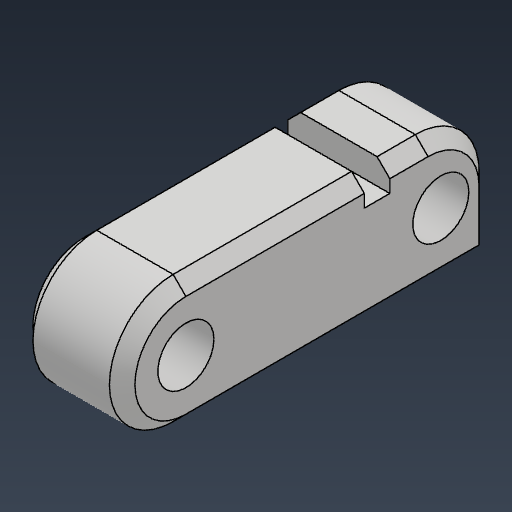
# Autodesk Inventor part: Chipanschlag L2.0
Saved by Autodesk Inventor 2023.1 (Build 271208000, 208)
## iProperties
Part Number: Chipanschlag L2.0
Material: Generisch
Document SubType Name: Modeling
Designer: rYan
Density: 1 g/cm^3
Appearance: Vorgabe
Author: rYan
Autodesk Inventor part; units mm, degrees
ref_plane "YZ Plane" through (0, 0, 0) normal (1, 0, 0) x (0, 1, 0)
ref_plane "XZ Plane" through (0, 0, 0) normal (0, 1, 0) x (-1, 0, 0)
ref_plane "XY Plane" through (0, 0, 0) normal (0, 0, 1) x (1, 0, 0)
sketch "Skizze1" plane through (0, 0, 0) normal (1, 0, 0) x (0, 1, 0)
  line L0 (0, 0) -> (-10, 0) construction
  circle A0 centre (0, 0) radius 1.1
  circle A1 centre (-10, 0) radius 1.1
  arc A2 (-10, 2.5) -> (-10, -2.5) centre (-10, 0) ccw
  line L1 (-10, -2.5) -> (2, -2.5)
  line L2 (-10, 2.5) -> (-0.5, 2.5)
  arc A3 (2, 0) -> (-0.5, 2.5) centre (-0.5, 0) ccw
  line L3 (2, 0) -> (2, -2.5)
  dimension "d0" = 10
  dimension "d1" = 2.2
  dimension "d2" = 2.2
  dimension "d3" = 2.5
  dimension "d8" = 2.5
  dimension "d9" = 2
  constraints: 8 end point, 4 centre point, 4 coincident, 4 point on circle, 4 tangent, 3 horizontal, 1 vertical
  measures "d0" distance of L0.start L0.end
  measures "d1" diameter of A0
  measures "d2" diameter of A1
  measures "d3" radius of A2
  measures "d8" radius of A3
  measures "d9" distance from line of L3 point (0, 0)
extrude "Extrusion1" add sketch "Skizze1" along normal mid plane 4
chamfer "Fase1" distance 0.5 angle 45 10 edges at (2, 1.2678, 1.7678) (2, -5.25, 2.5) (2, -12.5, 0) (2, -4, -2.5) (2, 2, -1.25) (-2, 1.2678, 1.7678) (-2, -5.25, 2.5) (-2, -12.5, 0) (-2, -4, -2.5) (-2, 2, -1.25)
sketch "Skizze5" plane through (-1.5, -10, 2.5) normal (0, 0, 1) x (1, 0, 0)
  line L0 (1.5, 14.9) -> (1.5, -5.4) projected
  line L1 (-1.3, 10) -> (4.3, 10) projected
  line L2 (3.5, 8) -> (-0.5, 8)
  line L3 (-0.5, 8) -> (-0.5, 7)
  line L4 (-0.5, 7) -> (3.5, 7)
  line L5 (3.5, 7) -> (3.5, 8)
  line L6 (3.5, 0) -> (3.5, 9.5) projected
  line L7 (-0.5, 9.5) -> (-0.5, 0) projected
  point P0 (1.5, 10)
  dimension "d26" = 1
  dimension "d27" = 2
  constraints: 8 end point, 2 collinear, 2 parallel, 1 horizontal, 1 perpendicular
  measures "d26" distance of L4.end L2.start
  measures "d27" distance between parallel lines of L1 L2
extrude "Extrusion4" cut sketch "Skizze5" against normal blind 1
pattern_linear "Rechteckige Anordnung1" [suppressed]
equation "\"d2\" = d1"
